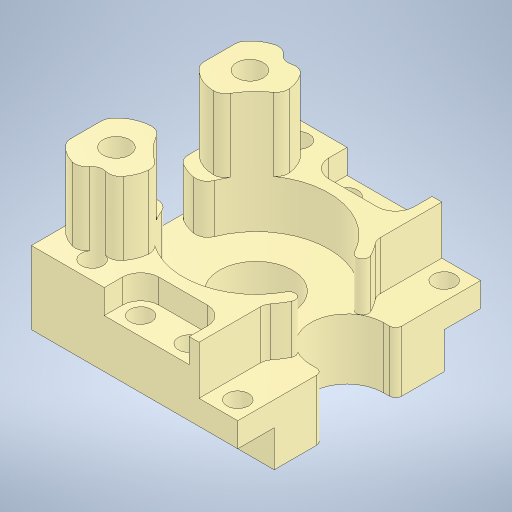
# Autodesk Inventor part: Spring Mount
Saved by Autodesk Inventor 2023.2 (Build 272271000, 271)
## iProperties
Created: 2024-03-24
Part Number: Spring Mount
Material: Nylon 6/6
Document SubType Name: Modeling
Designer: Nathan Cai
Density: 1.13 g/cm^3
Appearance: Nylon 6
Mass: 7.28213 g
Surface Area: 52.3259 cm^2
Volume: 6.44437 cm^3
Author: Nathan Cai
Autodesk Inventor part; units mm, degrees
ref_plane "YZ Plane" through (0, 0, 0) normal (1, 0, 0) x (0, 1, 0)
ref_plane "XZ Plane" through (0, 0, 0) normal (0, 1, 0) x (-1, 0, 0)
ref_plane "XY Plane" through (0, 0, 0) normal (0, 0, 1) x (1, 0, 0)
sketch "Sketch1" plane through (0, 0, 0) normal (0, 1, 0) x (-1, 0, 0)
  line L0 (-13.4938, 15.875) -> (13.4937, 15.875)
  line L1 (13.4937, 15.875) -> (13.4937, -15.875)
  line L2 (13.4937, -15.875) -> (-13.4938, -15.875)
  line L3 (-13.4938, -15.875) -> (-13.4938, 15.875)
  line L4 (-13.4938, 15.875) -> (13.4937, -15.875) construction
  line L5 (13.4937, 15.875) -> (-13.4938, -15.875) construction
  circle A0 centre (0, 0) radius 4.7625
  circle A1 centre (9.525, 8.7313) radius 6.35 construction
  line L6 (13.4937, 0) -> (-13.4938, 0) construction
  circle A2 centre (9.525, 8.7313) radius 1.7526
  circle A3 centre (9.525, -8.7312) radius 6.35 construction
  circle A4 centre (9.525, -8.7312) radius 1.7526
  dimension "d0" = 26.9875
  dimension "d1" = 31.75
  dimension "d2" = 9.525
  dimension "d3" = 12.7
  dimension "d4" = 3.5052
  dimension "d7" = 8.7312
  dimension "d8" = 3.9688
  constraints: 14 end point, 5 centre point, 4 midpoint, 2 coincident, 2 parallel, 2 symmetric about line, 1 horizontal, 1 perpendicular, 2 other
  measures "d0" distance of L1.end L2.end
  measures "d1" distance of L0.end L1.end
  measures "d2" diameter of A0
  measures "d3" diameter of A1
  measures "d4" diameter of A2
  measures "d7" distance from line of L6 A2.centre
  measures "d8" distance from line of L1 A2.centre
extrude "Extrusion1" add sketch "Sketch1" along normal blind 3.175
sketch "Sketch2" plane through (0, 3.175, 0) normal (0, 1, 0) x (1, 0, 0)
  circle A0 centre (0, 0) radius 9.525
  circle A1 centre (-9.525, 8.7312) radius 1.7526 projected
  circle A2 centre (-9.525, 8.7312) radius 6.35
  line L0 (13.4938, 15.875) -> (-13.4937, 15.875) projected
  line L1 (-13.4937, 15.875) -> (-13.4937, -15.875) projected
  line L2 (-13.4937, -15.875) -> (13.4938, -15.875) projected
  line L3 (13.4938, -15.875) -> (13.4938, 15.875) projected
  circle A3 centre (-9.525, 8.7312) radius 1.7526 projected
  circle A4 centre (-9.525, -8.7313) radius 1.7526 projected
  circle A5 centre (0, 0) radius 4.7625 projected
  circle A6 centre (-9.525, -8.7313) radius 6.35
  point P0 (-13.4937, 13.6882)
  point P1 (-13.4937, 3.7743)
  point P2 (-9.2207, 2.3885)
  point P3 (-3.1798, 8.9786)
  point P4 (-9.2207, -2.3885)
  point P5 (-13.4937, -3.7743)
  point P6 (-13.4937, -13.6882)
  point P7 (-3.1798, -8.9786)
  dimension "d9" = 19.05
  dimension "d10" = 12.7
  dimension "d11" = 12.7
  constraints: 3 centre point, 3 coincident
  measures "d9" diameter of A0
  measures "d10" diameter of A2
  measures "d11" diameter of A6
extrude "Extrusion2" add sketch "Sketch2" along normal blind 6.35 contours A0 A2 L1 L0 L3 L2 A6 | A0 A2 L1 | A6 L1 A0
sketch "Sketch3" plane through (0, 9.525, 0) normal (0, 1, 0) x (1, 0, 0)
  circle A0 centre (-9.525, -8.7313) radius 1.7526 projected
  circle A1 centre (-9.525, -8.7313) radius 4.699
  circle A2 centre (-9.525, 8.7312) radius 1.7526 projected
  circle A3 centre (-9.525, 8.7312) radius 4.699
  arc A4 (-13.4937, 3.7743) -> (-9.2207, 2.3885) centre (-9.525, 8.7312) ccw projected
  arc A5 (-9.2207, -2.3885) -> (-9.2207, 2.3885) centre (0, 0) ccw projected
  line L0 (-13.4937, 15.875) -> (-13.4937, 3.7743) projected
  circle A6 centre (-9.525, 8.7312) radius 1.7526 projected
  line L1 (-13.4937, -3.7743) -> (-13.4937, -15.875) projected
  arc A7 (-9.2207, -2.3885) -> (-13.4937, -3.7743) centre (-9.525, -8.7313) ccw projected
  arc A8 (-9.2207, -2.3885) -> (-9.2207, 2.3885) centre (0, 0) ccw projected
  circle A9 centre (-9.525, -8.7313) radius 1.7526 projected
  arc A10 (-13.4937, 3.7743) -> (-9.2207, 2.3885) centre (-9.525, 8.7312) ccw projected
  line L2 (-13.4937, -15.875) -> (13.4938, -15.875) projected
  line L3 (13.4938, -15.875) -> (13.4938, 15.875) projected
  line L4 (13.4938, 15.875) -> (-13.4937, 15.875) projected
  line L5 (-13.4937, 15.875) -> (-13.4937, 3.7743) projected
  arc A11 (-9.2207, -2.3885) -> (-13.4937, -3.7743) centre (-9.525, -8.7313) ccw projected
  line L6 (-13.4937, -3.7743) -> (-13.4937, -15.875) projected
  line L7 (-13.4937, -15.875) -> (13.4938, -15.875) projected
  line L8 (13.4938, -15.875) -> (13.4938, 15.875) projected
  line L9 (13.4938, 15.875) -> (-13.4937, 15.875) projected
  point P0 (-4.8568, -8.1937)
  point P1 (-8.5843, -4.1274)
  point P2 (-13.4937, -6.2154)
  point P3 (-13.4937, -11.2471)
  point P4 (-13.4937, 11.2471)
  point P5 (-13.4937, 6.2154)
  point P6 (-8.5843, 4.1274)
  point P7 (-4.8568, 8.1937)
  dimension "d14" = 9.398
  dimension "d15" = 9.398
  constraints: 2 centre point, 2 coincident
  measures "d14" diameter of A1
  measures "d15" diameter of A3
extrude "Extrusion3" add sketch "Sketch3" along normal blind 9.525 contours A1 L1 A5 | A5 A3 L0
sketch "Sketch4" plane through (0, 0, 0) normal (0, -1, 0) x (1, 0, 0)
  line L0 (-13.4937, -3.7743) -> (-13.4937, 3.7743) projected
  line L1 (-13.4937, 13.4938) -> (13.4938, 13.4937) construction
  line L2 (13.4938, 15.875) -> (13.4938, -15.875) projected
  line L3 (-13.4937, 15.875) -> (13.4938, 15.875) projected
  circle A0 centre (-7.9375, 13.4938) radius 1.4224
  circle A1 centre (-1.5875, 13.4937) radius 1.4224
  circle A2 centre (4.7625, 13.4937) radius 1.4224
  circle A3 centre (11.1125, 13.4937) radius 1.4224
  line L4 (-13.4937, -3.7743) -> (-13.4937, 3.7743) projected
  line L5 (-13.4937, 0) -> (13.4938, 0) construction
  line L6 (-13.4938, -13.4937) -> (13.4938, -13.4937) construction
  circle A4 centre (-7.9375, -13.4938) radius 1.4224
  circle A5 centre (-1.5875, -13.4938) radius 1.4224
  circle A6 centre (4.7625, -13.4937) radius 1.4224
  circle A7 centre (11.1125, -13.4937) radius 1.4224
  point P0 (0, 0)
  point P1 (-13.4937, 12.8557)
  point P2 (-13.4937, -4.6068)
  point P3 (-13.4937, 4.6068)
  dimension "d19" = 2.3813
  dimension "d20" = 2.8448
  dimension "d21" = 5.5563
  dimension "d24" = 6.35
  constraints: 8 centre point, 6 end point, 6 symmetric about line, 4 point on line, 2 midpoint, 1 horizontal, 1 parallel, 10 other
  measures "d19" distance between parallel lines of L3 L1
  measures "d20" diameter of A0
  measures "d21" distance from line of L0 A0.centre
  measures "d24" distance of A0.centre A1.centre
extrude "Extrusion4" cut sketch "Sketch4" against normal through all
sketch "Sketch5" plane through (0, 9.525, 0) normal (0, 1, 0) x (1, 0, 0)
  line L0 (13.4938, -15.875) -> (13.4938, 15.875) projected
  line L1 (13.4938, 0) -> (-13.4937, 0) construction
  line L2 (-13.4937, 15.875) -> (-13.4937, -15.875) projected
  line L3 (4.7625, -13.4937) -> (-1.5875, -13.4937) construction
  line L4 (4.7625, -11.1125) -> (-1.5875, -11.1125)
  line L5 (-1.5875, -15.875) -> (4.7625, -15.875)
  arc A0 (4.7625, -15.875) -> (4.7625, -11.1125) centre (4.7625, -13.4937) ccw
  arc A1 (-1.5875, -11.1125) -> (-1.5875, -15.875) centre (-1.5875, -13.4937) ccw
  line L6 (-13.4937, -15.875) -> (13.4938, -15.875) projected
  line L7 (7.1438, -13.4937) -> (-3.9687, -13.4937) construction
  line L8 (-3.9687, -13.4937) -> (-3.9687, -15.875)
  line L9 (-3.9687, -15.875) -> (7.1438, -15.875)
  line L10 (7.1438, -15.875) -> (7.1438, -13.4937)
  line L11 (4.7625, 13.4937) -> (-1.5875, 13.4937) construction
  line L12 (4.7625, 11.1125) -> (-1.5875, 11.1125)
  line L13 (-1.5875, 15.875) -> (4.7625, 15.875)
  arc A2 (4.7625, 11.1125) -> (4.7625, 15.875) centre (4.7625, 13.4937) ccw
  arc A3 (-1.5875, 15.875) -> (-1.5875, 11.1125) centre (-1.5875, 13.4937) ccw
  line L14 (7.1437, 13.4937) -> (-3.9688, 13.4937) construction
  line L15 (-3.9688, 13.4937) -> (-3.9688, 15.875)
  line L16 (-3.9688, 15.875) -> (7.1437, 15.875)
  line L17 (7.1437, 15.875) -> (7.1437, 13.4937)
  circle A4 centre (4.7625, -13.4937) radius 1.4224 projected
  circle A5 centre (-1.5875, -13.4937) radius 1.4224 projected
  point P0 (0, 0)
  point P1 (1.5875, -13.4937)
  point P2 (1.5875, 13.4937)
  point P3 (-3.9687, 13.4937)
  point P4 (-3.9687, -13.4937)
  point P5 (7.1438, -15.875)
  constraints: 34 end point, 11 symmetric about line, 9 point on circle, 5 tangent, 4 centre point, 3 midpoint, 3 parallel, 2 concentric, 2 horizontal, 2 point on line, 1 perpendicular, 2 other
extrude "Extrusion5" cut sketch "Sketch5" along normal blind 25.4 and the other way blind 3.175 contours A0 L5 A1 L4 | L10 L6 A0 | A1 L6 L8 | L12 A3 L13 A2 | A2 L16 L17 | L15 L16 A3 | A4 | A5
fillet "Fillet3" radius 1.5875 16 edges at (-4.8568, 14.2875, 8.1937) (-8.5843, 14.2875, 4.1274) (-13.4937, 14.2875, -11.2471) (-4.8568, 14.2875, -8.1937) (-8.5843, 14.2875, -4.1274) (-13.4937, 14.2875, 11.2471) (-13.4937, 14.2875, 6.2154) (-13.4937, 14.2875, -6.2154) (-9.2207, 6.35, 2.3885) (-9.2207, 6.35, -2.3885) (-13.4937, 6.35, -3.7743) (-13.4937, 6.35, 3.7743) (-6.8407, 14.2875, -12.5881) (-9.3583, 14.2875, -13.4273) (-9.3583, 14.2875, 13.4273) (-6.8407, 14.2875, 12.5881)
sketch "Sketch6" plane through (0, 9.525, 0) normal (0, 1, 0) x (1, 0, 0)
  line L0 (13.4938, -15.875) -> (13.4938, 15.875) projected
  circle A0 centre (0, 0) radius 11.1125
  line L1 (7.1438, -15.875) -> (13.4938, -15.875) projected
  line L2 (8.422, -15.875) -> (8.422, -7.2497)
  line L3 (0, 0) -> (11.1125, 0) construction
  line L4 (7.1438, -13.4937) -> (7.1438, -15.875) projected
  line L5 (8.422, 15.875) -> (8.422, 7.2497)
  line L6 (7.1437, 15.875) -> (7.1437, 13.4937) projected
  arc A1 (4.7625, 11.1125) -> (7.1437, 13.4937) centre (4.7625, 13.4937) ccw projected
  line L7 (4.7625, 11.1125) -> (-1.5875, 11.1125) projected
  arc A2 (-3.9687, 13.4937) -> (-1.5875, 11.1125) centre (-1.5875, 13.4937) ccw projected
  arc A3 (-4.8527, 9.2314) -> (-5.7879, 11.5799) centre (-9.525, 8.7312) ccw projected
  arc A4 (-5.5124, 7.7678) -> (-4.8527, 9.2314) centre (-6.4312, 9.0624) ccw projected
  arc A5 (-5.5124, -7.7678) -> (-5.5124, 7.7678) centre (0, 0) ccw projected
  arc A6 (-4.8527, -9.2314) -> (-5.5124, -7.7678) centre (-6.4312, -9.0624) ccw projected
  arc A7 (-5.7879, -11.5799) -> (-4.8527, -9.2314) centre (-9.525, -8.7313) ccw projected
  arc A8 (-1.5875, -11.1125) -> (-3.9687, -13.4937) centre (-1.5875, -13.4937) ccw projected
  line L8 (-1.5875, -11.1125) -> (4.7625, -11.1125) projected
  arc A9 (7.1438, -13.4937) -> (4.7625, -11.1125) centre (4.7625, -13.4937) ccw projected
  line L9 (7.1438, -13.4937) -> (7.1438, -15.875) projected
  line L10 (7.1438, -15.875) -> (13.4938, -15.875) projected
  line L11 (13.4938, -15.875) -> (13.4938, 15.875) projected
  line L12 (13.4938, 15.875) -> (7.1437, 15.875) projected
  line L13 (-3.9687, 13.4937) -> (-3.9688, 15.875) projected
  line L14 (-3.9688, 15.875) -> (-13.4937, 15.875) projected
  line L15 (-13.4937, 15.875) -> (-13.4937, 10.734) projected
  arc A10 (-13.1212, 11.7558) -> (-13.4937, 10.734) centre (-11.9062, 10.734) ccw projected
  arc A11 (-10.8055, 13.2524) -> (-13.1212, 11.7558) centre (-9.525, 8.7312) ccw projected
  arc A12 (-7.5183, 12.1345) -> (-9.0884, 12.6579) centre (-7.9375, 13.4938) ccw projected
  arc A13 (-10.6273, 2.4776) -> (-8.8729, 3.4638) centre (-10.3517, 4.041) ccw projected
  arc A14 (-8.2169, 4.8174) -> (-8.8729, 3.4638) centre (0, 0) ccw projected
  arc A15 (-9.6177, 4.0332) -> (-8.2169, 4.8174) centre (-9.5864, 5.6204) ccw projected
  arc A16 (-13.1212, 5.7067) -> (-9.6177, 4.0332) centre (-9.525, 8.7312) ccw projected
  arc A17 (-13.4937, 6.7285) -> (-13.1212, 5.7067) centre (-11.9062, 6.7285) ccw projected
  line L16 (-13.4937, 6.7285) -> (-13.4937, 4.6068) projected
  arc A18 (-13.4937, 4.6068) -> (-12.7, 3.232) centre (-11.9062, 4.6068) ccw projected
  arc A19 (-12.7, 3.232) -> (-10.6273, 2.4776) centre (-9.525, 8.7312) ccw projected
  arc A20 (-9.0884, -12.6579) -> (-7.5183, -12.1345) centre (-7.9375, -13.4938) ccw projected
  arc A21 (-13.1212, -11.7558) -> (-10.8055, -13.2524) centre (-9.525, -8.7313) ccw projected
  arc A22 (-13.4937, -10.734) -> (-13.1212, -11.7558) centre (-11.9062, -10.734) ccw projected
  line L17 (-13.4937, -10.734) -> (-13.4937, -15.875) projected
  line L18 (-13.4937, -15.875) -> (-3.9687, -15.875) projected
  line L19 (-3.9687, -15.875) -> (-3.9687, -13.4937) projected
  arc A23 (-8.8729, -3.4638) -> (-10.6273, -2.4776) centre (-10.3517, -4.041) ccw projected
  arc A24 (-10.6273, -2.4776) -> (-12.7, -3.232) centre (-9.525, -8.7313) ccw projected
  arc A25 (-12.7, -3.232) -> (-13.4937, -4.6068) centre (-11.9062, -4.6068) ccw projected
  line L20 (-13.4937, -4.6068) -> (-13.4937, -6.7285) projected
  arc A26 (-13.1212, -5.7067) -> (-13.4937, -6.7285) centre (-11.9062, -6.7285) ccw projected
  arc A27 (-9.6177, -4.0332) -> (-13.1212, -5.7067) centre (-9.525, -8.7313) ccw projected
  arc A28 (-8.2169, -4.8174) -> (-9.6177, -4.0332) centre (-9.5864, -5.6204) ccw projected
  arc A29 (-8.8729, -3.4638) -> (-8.2169, -4.8174) centre (0, 0) ccw projected
  arc A30 (-9.0884, 12.6579) -> (-10.8055, 13.2524) centre (-10.3729, 11.725) ccw projected
  arc A31 (-5.7879, 11.5799) -> (-7.5183, 12.1345) centre (-7.0505, 10.6175) ccw projected
  arc A32 (-7.5183, -12.1345) -> (-5.7879, -11.5799) centre (-7.0505, -10.6175) ccw projected
  arc A33 (-10.8055, -13.2524) -> (-9.0884, -12.6579) centre (-10.3729, -11.725) ccw projected
  point P0 (8.422, 15.875)
  point P1 (8.422, 7.2497)
  point P2 (3.9688, -14.6741)
  dimension "d42" = 22.225
  dimension "d43" = 1.2782
  constraints: 6 end point, 2 perpendicular, 2 point on circle, 2 symmetric about line, 1 centre point, 1 coincident, 1 point on line, 1 other
  measures "d42" diameter of A0
extrude "Extrusion6" cut sketch "Sketch6" against normal blind 6.35 contours L1 L2 A0 L5 L12 L0
fillet "Fillet4" radius 1.5875 2 edges at (8.422, 6.35, -7.2497) (8.422, 6.35, 7.2497)
sketch "Sketch7" plane through (0, 0, 0) normal (0, -1, 0) x (1, 0, 0)
  line L0 (13.4938, 15.875) -> (13.4938, -15.875) projected
  line L1 (-13.4938, -11.1125) -> (13.4938, -11.1125)
  line L2 (13.4938, -11.1125) -> (13.4938, 11.1125)
  line L3 (13.4938, 11.1125) -> (-13.4938, 11.1125)
  line L4 (-13.4938, 11.1125) -> (-13.4938, -11.1125)
  line L5 (-13.4938, -11.1125) -> (13.4938, 11.1125) construction
  line L6 (13.4938, -11.1125) -> (-13.4938, 11.1125) construction
  line L7 (-13.4937, 15.875) -> (13.4938, 15.875) projected
  circle A0 centre (0, 0) radius 8 construction
  circle A1 centre (0, 0) radius 9.5 construction
  line L8 (0, 0) -> (0, 9.525) construction
  arc A2 (-5.5124, -7.7678) -> (-5.5124, 7.7678) centre (0, 0) ccw projected
  line L9 (0, 0) -> (-6.7352, 6.7352) construction
  arc A3 (-8.8729, -3.4638) -> (-8.8729, 3.4638) centre (0, 0) ccw projected
  line L10 (-5.6569, 5.6569) -> (-6.7352, 6.7352) construction
  line L11 (-3.8891, 7.4246) -> (-4.9674, 8.503)
  line L12 (-8.503, 4.9674) -> (-7.4246, 3.8891)
  arc A4 (-7.4246, 3.8891) -> (-3.8891, 7.4246) centre (-5.6569, 5.6569) ccw
  arc A5 (-4.9674, 8.503) -> (-8.503, 4.9674) centre (-6.7352, 6.7352) ccw
  circle A6 centre (-9.525, 8.7313) radius 1.7526 projected
  arc A7 (-8.503, -4.9674) -> (-4.9674, -8.503) centre (-6.7352, -6.7352) ccw
  line L13 (-4.9674, -8.503) -> (-3.8891, -7.4246)
  line L14 (-7.4246, -3.8891) -> (-8.503, -4.9674)
  arc A8 (-3.8891, -7.4246) -> (-7.4246, -3.8891) centre (-5.6569, -5.6569) ccw
  arc A9 (4.9674, -8.503) -> (8.503, -4.9674) centre (6.7352, -6.7352) ccw
  line L15 (8.503, -4.9674) -> (7.4246, -3.8891)
  line L16 (3.8891, -7.4246) -> (4.9674, -8.503)
  arc A10 (7.4246, -3.8891) -> (3.8891, -7.4246) centre (5.6569, -5.6569) ccw
  arc A11 (8.503, 4.9674) -> (4.9674, 8.503) centre (6.7352, 6.7352) ccw
  line L17 (4.9674, 8.503) -> (3.8891, 7.4246)
  line L18 (7.4246, 3.8891) -> (8.503, 4.9674)
  arc A12 (3.8891, 7.4246) -> (7.4246, 3.8891) centre (5.6569, 5.6569) ccw
  circle A13 centre (11.1125, 13.4937) radius 1.4224 projected
  circle A14 centre (-1.5875, 13.4937) radius 1.4224 projected
  circle A15 centre (-1.5875, -13.4938) radius 1.4224 projected
  circle A16 centre (11.1125, -13.4937) radius 1.4224 projected
  circle A17 centre (-7.9375, -13.4938) radius 1.4224 projected
  circle A18 centre (-7.9375, 13.4938) radius 1.4224 projected
  circle A19 centre (4.7625, 13.4937) radius 1.4224 projected
  circle A20 centre (4.7625, -13.4937) radius 1.4224 projected
  line L19 (13.4938, -15.875) -> (-13.4937, -15.875) projected
  line L20 (13.4938, 15.875) -> (13.4938, -15.875) projected
  line L21 (-13.4937, 15.875) -> (13.4938, 15.875) projected
  line L22 (-13.4937, -15.875) -> (-13.4937, 15.875) projected
  circle A21 centre (-9.525, -8.7312) radius 1.7526 projected
  circle A22 centre (-9.525, 8.7313) radius 1.7526 projected
  circle A23 centre (0, 0) radius 4.7625 projected
  point P0 (-6.196, 6.196)
  point P1 (-7.7932, -9.0003)
  point P2 (-9.2206, -7.0053)
  point P3 (-9.2206, 7.0053)
  point P4 (-7.7932, 9.0003)
  dimension "d46" = 16
  dimension "d45" = 4.7625
  dimension "d47" = 19
  dimension "d48" = 45
  dimension "d51" = 360
  dimension "d53" = 2.5
  constraints: 36 end point, 18 point on circle, 9 centre point, 4 tangent, 3 midpoint, 3 parallel, 2 coincident, 2 point on line, 1 collinear, 1 horizontal, 1 perpendicular, 1 vertical, 44 other
  measures "d45" distance between parallel lines of L7 L3
  measures "d47" diameter of A1
  measures "d48" angle of L8 L9
  measures "d53" radius of A5
extrude "Extrusion7" add sketch "Sketch7" along normal blind 4.7625 contours L0 L1 L4 L3
fillet "Fillet5" radius 6.35 4 edges at (-9.2206, -2.3813, -7.0053) (-7.7932, -2.3813, -9.0003) (-9.2206, -2.3813, 7.0053) (-7.7932, -2.3813, 9.0003)
sketch "Sketch8" plane through (0, -4.7625, 0) normal (0, -1, 0) x (1, 0, 0)
  line L0 (15.0813, 0) -> (11.9063, 0) construction
  line L1 (13.4938, -11.1125) -> (13.4938, 11.1125) projected
  line L2 (15.0813, 4.7625) -> (11.9063, 4.7625)
  line L3 (11.9063, -4.7625) -> (15.0813, -4.7625)
  arc A0 (15.0813, -4.7625) -> (15.0813, 4.7625) centre (15.0813, 0) ccw
  arc A1 (11.9063, 4.7625) -> (11.9063, -4.7625) centre (11.9063, 0) ccw
  point P0 (0, 0)
  point P1 (13.4938, 0)
  point P2 (13.4938, -4.7625)
  point P3 (13.4938, 4.7625)
  dimension "d57" = 9.525
  dimension "d58" = 3.175
  constraints: 8 end point, 4 point on circle, 4 tangent, 2 centre point, 2 midpoint, 1 horizontal, 1 parallel
  measures "d57" diameter of A1
  measures "d58" distance of L0.end L0.start
extrude "Extrusion8" cut sketch "Sketch8" against normal through all contours L3 A1 L2 L1
fillet "Fillet6" radius 0.7937 6 edges at (8.8106, 6.35, -3.6192) (8.8106, 6.35, 3.6192) (10.1865, 6.35, -4.4411) (10.1865, 6.35, 4.4411) (13.4938, -0.7937, 4.7625) (13.4938, -0.7937, -4.7625)
equation "\"d11\" = d10"
body "Solid1"
